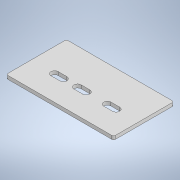
# Autodesk Inventor part: back
Saved by Autodesk Inventor 2021 (Build 250183000, 183)
## iProperties
Created: 2025-12-27
Part Number: back
Material: Generic
Description: FreeCAD Model
Document SubType Name: Sheet Metal
Designer: Ignacio
Authority: Unknown
Density: 1 g/cm^3
Appearance: Default
Sheet Metal Rule: Default
Sending System: FreeCAD
Preprocessor: Open CASCADE STEP processor 7.6
Title: Open CASCADE Shape Model
Autodesk Inventor part; units mm, degrees
ref_plane "YZ Plane" through (0, 0, 0) normal (1, 0, 0) x (0, 1, 0)
ref_plane "XZ Plane" through (0, 0, 0) normal (0, 1, 0) x (-1, 0, 0)
ref_plane "XY Plane" through (0, 0, 0) normal (0, 0, 1) x (1, 0, 0)
sketch "Sketch2" plane through (0, 0, 0) normal (0, 1, 0) x (-1, 0, 0)
  line L0 (0, 0) -> (125.1, 0)
  line L1 (125.1, 0) -> (125.1, -70.1)
  line L2 (125.1, -70.1) -> (0, -70.1)
  line L3 (0, -70.1) -> (0, 0)
  dimension "d5" = 70.1
  dimension "d6" = 125.1
  constraints: 8 end point, 2 parallel, 1 horizontal, 1 perpendicular
  measures "d5" distance of L0.end L1.end
  measures "d6" distance of L1.end L2.end
extrude "Extrusion2" add sketch "Sketch2" along normal blind 4
fillet "Fillet1" radius 2 4 edges at (-125.1, 2, 0) (-125.1, 2, -70.1) (0, 2, 0) (0, 2, -70.1)
sketch "Sketch4" plane through (0, 0, 0) normal (0, -1, 0) x (1, 0, 0)
  line L0 (-60.7951, -25.715) -> (-60.7951, -33.115) projected
  line L1 (-60.7951, -33.115) -> (-70.9551, -33.115) projected
  line L2 (-70.9551, -25.715) -> (-70.9551, -33.115) projected
  line L3 (-60.7951, -25.715) -> (-70.9551, -25.715) projected
  line L4 (-70.2151, -31.515) -> (-66.6151, -31.515) projected
  line L5 (-66.6151, -31.515) -> (-66.6151, -26.315) projected
  line L6 (-66.6151, -26.315) -> (-70.2151, -26.315) projected
  line L7 (-70.2151, -26.315) -> (-70.2151, -31.515) projected
  line L8 (-65.1351, -31.515) -> (-61.5351, -31.515) projected
  line L9 (-61.5351, -31.515) -> (-61.5351, -26.315) projected
  line L10 (-61.5351, -26.315) -> (-65.1351, -26.315) projected
  line L11 (-65.1351, -26.315) -> (-65.1351, -31.515) projected
  line L12 (-87.4551, -25.715) -> (-87.4551, -33.115) projected
  line L13 (-87.4551, -33.115) -> (-97.6151, -33.115) projected
  line L14 (-97.6151, -25.715) -> (-97.6151, -33.115) projected
  line L15 (-87.4551, -25.715) -> (-97.6151, -25.715) projected
  line L16 (-96.8751, -31.515) -> (-93.2751, -31.515) projected
  line L17 (-93.2751, -31.515) -> (-93.2751, -26.315) projected
  line L18 (-93.2751, -26.315) -> (-96.8751, -26.315) projected
  line L19 (-96.8751, -26.315) -> (-96.8751, -31.515) projected
  line L20 (-91.7951, -31.515) -> (-88.1951, -31.515) projected
  line L21 (-88.1951, -31.515) -> (-88.1951, -26.315) projected
  line L22 (-88.1951, -26.315) -> (-91.7951, -26.315) projected
  line L23 (-91.7951, -26.315) -> (-91.7951, -31.515) projected
  line L24 (-26.0551, -25.715) -> (-26.0551, -33.115) projected
  line L25 (-26.0551, -33.115) -> (-36.2151, -33.115) projected
  line L26 (-36.2151, -25.715) -> (-36.2151, -33.115) projected
  line L27 (-26.0551, -25.715) -> (-36.2151, -25.715) projected
  line L28 (-35.4751, -31.515) -> (-31.8751, -31.515) projected
  line L29 (-31.8751, -31.515) -> (-31.8751, -26.315) projected
  line L30 (-31.8751, -26.315) -> (-35.4751, -26.315) projected
  line L31 (-35.4751, -26.315) -> (-35.4751, -31.515) projected
  line L32 (-30.3951, -31.515) -> (-26.7951, -31.515) projected
  line L33 (-26.7951, -31.515) -> (-26.7951, -26.315) projected
  line L34 (-26.7951, -26.315) -> (-30.3951, -26.315) projected
  line L35 (-30.3951, -26.315) -> (-30.3951, -31.515) projected
  line L36 (-101.8351, -28.915) -> (-21.8351, -28.915) construction
  line L37 (-97.6351, -33.115) -> (-26.0351, -33.115) construction
  line L38 (-26.0351, -24.715) -> (-97.6351, -24.715) construction
  arc A0 (-97.6351, -24.715) -> (-97.6351, -33.115) centre (-97.6351, -28.915) ccw
  arc A1 (-26.0351, -33.115) -> (-26.0351, -24.715) centre (-26.0351, -28.915) ccw
  line L39 (-97.6151, -25.715) -> (-97.6151, -10.355) construction
  line L40 (-26.0551, -25.715) -> (-26.0551, -14.2023) construction
  line L41 (-101.8351, -28.915) -> (-101.8351, -10.355) construction
  line L42 (-101.8351, -10.355) -> (-97.6151, -10.355) construction
  line L43 (-26.0551, -14.2023) -> (-21.8351, -14.2023) construction
  line L44 (-21.8351, -14.2023) -> (-21.8351, -28.915) construction
  line L45 (-101.8351, -28.915) -> (-83.2351, -28.915) construction
  line L46 (-97.6351, -33.115) -> (-87.4351, -33.115)
  line L47 (-87.4351, -24.715) -> (-97.6351, -24.715)
  arc A2 (-97.6351, -24.715) -> (-97.6351, -33.115) centre (-97.6351, -28.915) ccw
  arc A3 (-87.4351, -33.115) -> (-87.4351, -24.715) centre (-87.4351, -28.915) ccw
  line L48 (-75.1751, -28.915) -> (-56.5751, -28.915) construction
  line L49 (-70.9751, -33.115) -> (-60.7751, -33.115)
  line L50 (-60.7751, -24.715) -> (-70.9751, -24.715)
  arc A4 (-70.9751, -24.715) -> (-70.9751, -33.115) centre (-70.9751, -28.915) ccw
  arc A5 (-60.7751, -33.115) -> (-60.7751, -24.715) centre (-60.7751, -28.915) ccw
  line L51 (-40.4351, -28.915) -> (-21.8351, -28.915) construction
  line L52 (-36.2351, -33.115) -> (-26.0351, -33.115)
  line L53 (-26.0351, -24.715) -> (-36.2351, -24.715)
  arc A6 (-36.2351, -24.715) -> (-36.2351, -33.115) centre (-36.2351, -28.915) ccw
  arc A7 (-26.0351, -33.115) -> (-26.0351, -24.715) centre (-26.0351, -28.915) ccw
  point P0 (0, 0)
  point P1 (-61.8351, -28.915)
  point P2 (-92.5351, -28.915)
  point P3 (-65.8751, -28.915)
  point P4 (-31.1351, -28.915)
  point P5 (-97.6351, -24.715)
  point P6 (-26.0351, -33.115)
  point P7 (-26.0351, -24.715)
  dimension "d10" = 80
  dimension "d11" = 0
  dimension "d12" = 1
  dimension "d13" = 4.22
  dimension "d14" = 4.22
  dimension "d15" = 4.22
  dimension "d16" = 4.22
  dimension "d17" = 4.22
  constraints: 44 end point, 24 point on circle, 17 tangent, 15 point on line, 8 centre point, 6 parallel, 4 midpoint, 2 horizontal, 2 perpendicular, 2 vertical, 1 collinear
  measures "d10" distance of L36.start L36.end
  measures "d11" distance between parallel lines of L37 L13
  measures "d12" distance between parallel lines of L38 L15
  measures "d13" distance from line of L36.start L14
  measures "d14" distance from line of L45.end L12
  measures "d15" distance from line of L2 L48.start
  measures "d16" distance from line of L48.end L0
  measures "d17" distance from line of L26 L51.start
extrude "Extrusion3" cut sketch "Sketch4" against normal blind 10 contours L3 L2 L49 A4 L50 A5 L0 | L0 L1 L2 L3 | L7 L6 L5 L4 | L11 L10 L9 L8 | L15 L14 L46 A0 L47 A3 L12 | L12 L13 L14 L15 | L19 L18 L17 L16 | L23 L22 L21 L20 | L27 L26 L52 A6 L53 A1 L24 | L24 L25 L26 L27 | L31 L30 L29 L28 | L35 L34 L33 L32
equation "\"d14\" = d13"
equation "\"d15\" = d14"
equation "\"d16\" = d15"
equation "\"d17\" = d16"
equation "\"BendRadius\" = Thickness"
equation "\"BendReliefWidth\" = Thickness"
equation "\"BendReliefDepth\" = 0.5 * Thickness"
equation "\"CornerReliefSize\" = 4 * Thickness"
equation "\"MinimumRemnant\" = 2 * Thickness"
equation "\"TransitionRadius\" = BendRadius"
equation "\"JacobiRadiusSize\" = Thickness"
equation "\"GapSize\" = Thickness"
equation "\"Thickness\" = 0.5"
body "Solid2"
